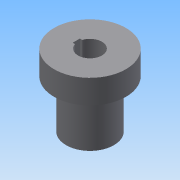
# Autodesk Inventor part: Колесо
Saved by Autodesk Inventor 2013 (Build 170138000, 138)
## iProperties
Created: 2018-03-30
Part Number: Колесо
Material: Типовые
Document SubType Name: Modeling
Designer: User
Density: 1 g/cm^3
Author: User
Autodesk Inventor part; units mm, degrees
ref_plane "YZ Plane" through (0, 0, 0) normal (1, 0, 0) x (0, 1, 0)
ref_plane "XZ Plane" through (0, 0, 0) normal (0, 1, 0) x (-1, 0, 0)
ref_plane "XY Plane" through (0, 0, 0) normal (0, 0, 1) x (1, 0, 0)
sketch "Эскиз1" plane through (0, 0, 0) normal (0, 0, 1) x (1, 0, 0)
  circle A0 centre (0, 0) radius 30
  dimension "d0" = 60
  constraints: 1 centre point, 1 coincident
  measures "d0" diameter of A0
extrude "Выдавливание1" add sketch "Эскиз1" against normal blind 20
sketch "Эскиз2" plane through (0, 0, -20) normal (0, 0, -1) x (-1, 0, 0)
  circle A0 centre (0, 0) radius 30 projected
  circle A1 centre (0, 0) radius 20
  dimension "d3" = 40
  constraints: 1 centre point, 1 coincident
  measures "d3" diameter of A1
extrude "Выдавливание2" add sketch "Эскиз2" along normal blind 40 contours A1
sketch "Эскиз3" plane through (0, 0, -60) normal (0, 0, -1) x (-1, 0, 0)
  circle A0 centre (0, 0) radius 20 projected
  arc A1 (9.5394, 3) -> (9.5394, -3) centre (0, 0) ccw
  line L0 (9.5394, 3) -> (11.5, 3)
  line L1 (11.5, 3) -> (11.5, -3)
  line L2 (11.5, -3) -> (9.5394, -3)
  dimension "d6" = 20
  dimension "d8" = 11.5
  dimension "d9" = 3
  dimension "d10" = 3
  constraints: 6 end point, 2 perpendicular, 2 point on circle, 1 centre point, 1 coincident, 1 horizontal
  measures "d6" diameter of A1
  measures "d8" distance from line of L1 A0.centre
  measures "d9" distance from line of L0 A0.centre
  measures "d10" distance from line of L2 A0.centre
extrude "Выдавливание3" cut sketch "Эскиз3" against normal through all contours L0 L1 L2 A1
fillet "Сопряжение2" radius 5 1 edges at (20, 0, -20)
